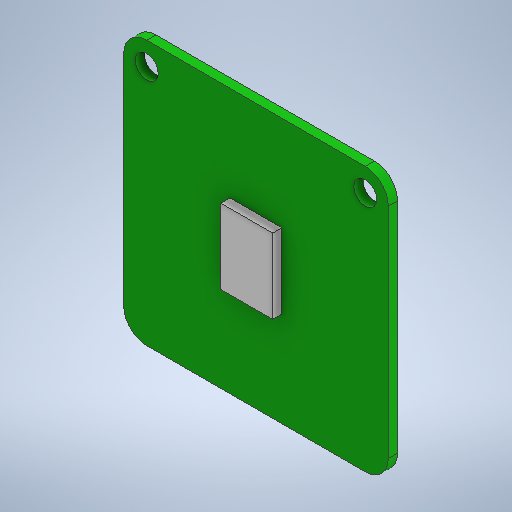
# Autodesk Inventor part: Encoder
Saved by Autodesk Inventor 2025.1 (Build 291241000, 241)
## iProperties
Created: 2025-10-26
Part Number: Encoder
Material: Generic
Document SubType Name: Modeling
Designer: paeze
Density: 1 g/cm^3
Appearance: Default
Author: paeze
Autodesk Inventor part; units mm, degrees
ref_plane "YZ Plane" through (0, 0, 0) normal (1, 0, 0) x (0, 1, 0)
ref_plane "XZ Plane" through (0, 0, 0) normal (0, 1, 0) x (-1, 0, 0)
ref_plane "XY Plane" through (0, 0, 0) normal (0, 0, 1) x (1, 0, 0)
sketch "Sketch1" plane through (0, 0, 0) normal (0, 0, 1) x (1, 0, 0)
  line L0 (-10.7511, 9.0038) -> (12.2489, 9.0038)
  line L1 (12.2489, 9.0038) -> (12.2489, -13.9962)
  line L2 (12.2489, -13.9962) -> (-10.7511, -13.9962)
  line L3 (-10.7511, -13.9962) -> (-10.7511, 9.0038)
  point P0 (0, 0)
  dimension "d0" = 23
  dimension "d1" = 23
  constraints: 8 end point, 2 parallel, 1 horizontal, 1 perpendicular
  measures "d0" distance of L1.end L2.end
  measures "d1" distance of L0.end L1.end
extrude "Extrusion1" add sketch "Sketch1" along normal blind 0.8
fillet "Fillet1" radius 2 4 edges at (12.2489, 9.0038, 0.4) (-10.7511, 9.0038, 0.4) (12.2489, -13.9962, 0.4) (-10.7511, -13.9962, 0.4)
sketch "Sketch2" plane through (0, 0, 0.8) normal (0, 0, 1) x (1, 0, 0)
  arc A0 (-8.7511, 9.0038) -> (-10.7511, 7.0038) centre (-8.7511, 7.0038) ccw projected
  circle A1 centre (-8.7511, 7.0038) radius 1
  arc A2 (12.2489, 7.0038) -> (10.2489, 9.0038) centre (10.2489, 7.0038) ccw projected
  circle A3 centre (10.2489, 7.0038) radius 1
  point P0 (0, 0)
  dimension "d5" = 2
  dimension "d6" = 2
  constraints: 2 centre point, 2 coincident
  measures "d5" diameter of A1
  measures "d6" diameter of A3
extrude "Extrusion2" cut sketch "Sketch2" against normal blind 0.8
sketch "Sketch3" plane through (0, 0, 0.8) normal (0, 0, 1) x (1, 0, 0)
  line L0 (10.2489, 9.0038) -> (-8.7511, 9.0038) projected
  line L1 (-8.7511, -13.9962) -> (10.2489, -13.9962) projected
  line L2 (0.7489, 9.0038) -> (10.2489, 9.0038)
  line L3 (10.2489, 9.0038) -> (10.2489, -13.9962)
  line L4 (10.2489, -13.9962) -> (0.7489, -13.9962)
  line L5 (0.7489, -13.9962) -> (0.7489, 9.0038)
  line L6 (2.9989, -5.7462) -> (-1.5011, -5.7462)
  line L7 (-1.5011, -5.7462) -> (-1.5011, 0.7538)
  line L8 (-1.5011, 0.7538) -> (2.9989, 0.7538)
  line L9 (2.9989, 0.7538) -> (2.9989, -5.7462)
  line L10 (2.9989, -5.7462) -> (-1.5011, 0.7538) construction
  line L11 (-1.5011, -5.7462) -> (2.9989, 0.7538) construction
  point P0 (0, 0)
  point P1 (0.7489, -2.4962)
  dimension "d9" = 4.5
  dimension "d10" = 6.5
  constraints: 20 end point, 4 midpoint, 4 parallel, 2 horizontal, 2 perpendicular
  measures "d9" distance of L7.end L8.end
  measures "d10" distance of L6.end L7.end
extrude "Extrusion3" add sketch "Sketch3" along normal blind 0.8 contours L8 L9 L6 L5 | L5 L6 L7 L8
body "Solid1"
